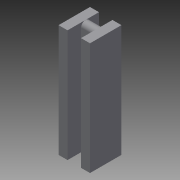
# Autodesk Inventor part: Cable Sliding Assistor
Saved by Autodesk Inventor 2015 (Build 190159000, 159)
## iProperties
Created: 2016-05-27
Part Number: Cable Sliding Assistor
Material: Generic
Document SubType Name: Modeling
Designer: Toby
Density: 1 g/cm^3
Appearance: Default
Author: Toby
Autodesk Inventor part; units mm, degrees
ref_plane "YZ Plane" through (0, 0, 0) normal (1, 0, 0) x (0, 1, 0)
ref_plane "XZ Plane" through (0, 0, 0) normal (0, 1, 0) x (-1, 0, 0)
ref_plane "XY Plane" through (0, 0, 0) normal (0, 0, 1) x (1, 0, 0)
sketch "Sketch1" plane through (0, 0, 0) normal (0, 0, 1) x (1, 0, 0)
  line L0 (-9.1579, 2.8421) -> (-7.1579, 2.8421)
  line L1 (-7.1579, 2.8421) -> (-7.1579, -1.1579)
  line L2 (-7.1579, -1.1579) -> (-9.1579, -1.1579)
  line L3 (-9.1579, -1.1579) -> (-9.1579, 2.8421)
  line L4 (-9.1579, 0.8421) -> (-2.1579, 0.8421)
  line L5 (-2.1579, 0.8421) -> (-2.1579, -1.1579)
  line L6 (-2.1579, -1.1579) -> (-9.1579, -1.1579)
  line L7 (-9.1579, -1.1579) -> (-9.1579, 0.8421)
  line L8 (-2.1579, -1.1579) -> (-4.1579, -1.1579)
  line L9 (-4.1579, -1.1579) -> (-4.1579, 2.8421)
  line L10 (-4.1579, 2.8421) -> (-2.1579, 2.8421)
  line L11 (-2.1579, 2.8421) -> (-2.1579, -1.1579)
  line L12 (-9.1579, 0.8421) -> (-7.1579, 0.8421)
  line L13 (-7.1579, 0.8421) -> (-7.1579, -4.1579)
  line L14 (-7.1579, -4.1579) -> (-9.1579, -4.1579)
  line L15 (-9.1579, -4.1579) -> (-9.1579, 0.8421)
  line L16 (-2.1579, 0.8421) -> (-4.1579, 0.8421)
  line L17 (-4.1579, 0.8421) -> (-4.1579, -4.1579)
  line L18 (-4.1579, -4.1579) -> (-2.1579, -4.1579)
  line L19 (-2.1579, -4.1579) -> (-2.1579, 0.8421)
  point P0 (0, 0)
  dimension "d0" = 2
  dimension "d1" = 2
  dimension "d2" = 3
  dimension "d3" = 3
  dimension "d4" = 2
  dimension "d5" = 2
  constraints: 40 end point, 10 parallel, 5 horizontal, 5 perpendicular, 5 point on line, 1 midpoint
  measures "d0" distance of L0.start L0.end
  measures "d1" distance of L9.end L10.end
  measures "d2" distance between parallel lines of L9 L1
  measures "d3" distance between parallel lines of L14 L6
  measures "d4" distance between parallel lines of L6 L4
  measures "d5" distance between parallel lines of L4 L0
extrude "Extrusion1" add sketch "Sketch1" along normal blind 25
fillet "Fillet1" radius 1 2 edges at (-5.6579, 0.8421, 25) (-5.6579, -1.1579, 25)
fillet "Fillet2" radius 1 2 edges at (-5.6579, 0.8421, 0) (-5.6579, -1.1579, 0)
body "Solid1"
